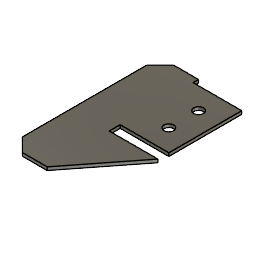
GPL H300 to 175G19_ (Autodesk Fusion 360 design; units mm, degrees)
Autodesk Fusion 360 part; units mm, degrees
sketch "スケッチ1" plane through (0, 0, 0) normal (0, 0, 1) x (1, 0, 0)
  line L0 (-9.5, 140) -> (-80.5, 140)
  line L1 (-80.5, 140) -> (-80.5, -140)
  line L2 (-80.5, -140) -> (-9.5, -140)
  line L3 (80.5, -5) -> (80.5, 130)
  line L4 (-9.5, 140) -> (-9.5, 130)
  line L5 (-9.5, 130) -> (80.5, 130)
  line L6 (-80.5, -140) -> (-9.5, -140) construction
  line L7 (80.5, -25) -> (-9.5, -140)
  line L8 (80.5, -25) -> (-9.5, -25)
  line L9 (-9.5, -25) -> (-9.5, -5)
  line L10 (-9.5, -5) -> (80.5, -5)
  line L11 (-80.5, 140) -> (2.875, -5) construction
  line L12 (14.375, -25) -> (42.3815, -73.707) construction
  line L13 (74.75, 130) -> (-2.875, -5) construction
  line L14 (-9.5, -16.5217) -> (-80.5, -140) construction
  dimension "d2" = 280
  dimension "d5" = 71
  dimension "d7" = 90
  dimension "d8" = 20
  constraint horizontal L0
  constraint perpendicular L0 L1
  constraint parallel L0 L2
  constraint parallel L1 L3
  constraint coincident origin L13
  constraint coincident origin L11
  constraint vertical L4
  constraint horizontal L5
  constraint coincident L5 L13.start
  constraint perpendicular L1 L6
  constraint coincident L7 L12.end
  constraint horizontal L8
  constraint vertical L9
  constraint horizontal L10
  constraint coincident L10 L11.end
  constraint coincident L8 L12.start
  constraint collinear L11 L12
  constraint coincident L10 L13.end
  constraint coincident L9 L14.start
  constraint collinear L13 L14
  measures "d2" distance of L0.end L1.end
  measures "d5" distance of L1.end L2.end
  measures "d7" distance of L7.start L8.end
  measures "d8" distance of L7.start L3.start
extrude "押し出し1" add sketch "スケッチ1" along normal blind 6
chamfer "面取り1" distance 25 angle 45 2 edges at (-80.5, -140, 3) (-80.5, 140, 3)
sketch "スケッチ2" plane through (0, 0, 6) normal (0, 0, 1) x (-1, 0, 0)
  line L0 (55.5, -140) -> (80.5, -115)
  line L1 (80.5, -115) -> (80.5, 115)
  line L2 (80.5, 115) -> (55.5, 140)
  line L3 (55.5, 140) -> (9.5, 140)
  line L4 (9.5, 140) -> (-80.5, 25)
  line L5 (-80.5, 25) -> (9.5, 25)
  line L6 (9.5, 25) -> (9.5, 5)
  line L7 (9.5, 5) -> (-80.5, 5)
  line L8 (-80.5, 5) -> (-80.5, -130)
  line L9 (-80.5, -130) -> (9.5, -130)
  line L10 (9.5, -130) -> (9.5, -140)
  line L11 (9.5, -140) -> (55.5, -140)
  line L12 (-80.5, -130) -> (-40.5, -130) construction
  line L13 (-40.5, -130) -> (-40.5, -90) construction
  line L14 (-40.5, -90) -> (-80.5, -90) construction
  line L15 (-80.5, -90) -> (-80.5, -130) construction
  line L16 (-40.5, -90) -> (-40.5, -35) construction
  point P0 (-40.5, -90)
  point P1 (-40.5, -35)
  dimension "d12" = 40
  dimension "d13" = 40
  dimension "d14" = 55
  constraint horizontal L12
  constraint vertical L13
  constraint horizontal L14
  constraint vertical L15
  constraint coincident L8.end L9.start
  constraint perpendicular L14 L16
  constraint coincident P0 L13.end
  constraint coincident P1 L16.end
  measures "d12" distance of L8.end L12.end
  measures "d13" distance of L8.end L14.end
  measures "d14" distance of P0 P1
hole "穴1" at (40.5, 90, 6) at (40.5, 35, 6) direction (0, 0, -1) diameter 18 end through all
equation "d5 = 25 mm + 46 mm"
